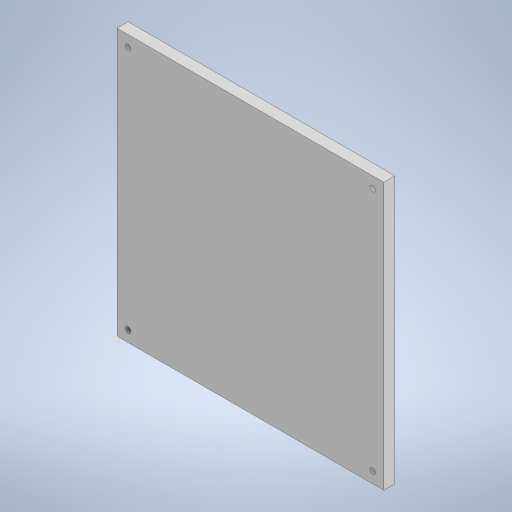
# Autodesk Inventor part: 3d_enclosure_2_19_top_1
Saved by Autodesk Inventor 2024 (Build 280153000, 153)
## iProperties
Created: 2024-02-19
Part Number: 3d_enclosure_2_19_top_1
Material: Generic
Document SubType Name: Modeling
Designer: jtw4137
Density: 1 g/cm^3
Appearance: Default
Author: jtw4137
Autodesk Inventor part; units mm, degrees
ref_plane "YZ Plane" through (0, 0, 0) normal (1, 0, 0) x (0, 1, 0)
ref_plane "XZ Plane" through (0, 0, 0) normal (0, 1, 0) x (-1, 0, 0)
ref_plane "XY Plane" through (0, 0, 0) normal (0, 0, 1) x (1, 0, 0)
sketch "Sketch1" plane through (0, 0, 0) normal (0, 0, 1) x (1, 0, 0)
  line L0 (0, 0) -> (120, 0)
  line L1 (120, 0) -> (120, 120)
  line L2 (120, 120) -> (0, 120)
  line L3 (0, 120) -> (0, 0)
  dimension "d0" = 120
  dimension "d1" = 120
  dimension "d2" = 120
  constraints: 8 end point, 2 perpendicular, 1 horizontal
  measures "d0" distance of L0.start L0.end
  measures "d1" distance of L0.end L1.end
  measures "d2" distance of L1.end L2.end
extrude "Extrusion1" add sketch "Sketch1" along normal blind 5
sketch "Sketch3" plane through (0, 0, 5) normal (0, 0, 1) x (1, 0, 0)
  line L0 (120, 120) -> (0, 120) projected
  line L1 (0, 120) -> (5, 120)
  line L2 (5, 120) -> (5, 115)
  point P0 (0, 0)
  dimension "d7" = 5
  dimension "d8" = 5
  constraints: 4 end point, 1 perpendicular, 1 point on line
  measures "d7" distance of L0.end L1.end
  measures "d8" distance of L1.end L2.end
hole "Hole1" at (5, 115, 5) direction (0, 0, -1) diameter 2.5 depth 38.1 tip angle 118
sketch "Sketch4" plane through (0, 0, 5) normal (0, 0, 1) x (1, 0, 0)
  line L0 (0, 120) -> (0, 0) projected
  line L1 (0, 0) -> (5, 0)
  line L2 (0, 0) -> (120, 0) projected
  line L3 (5, 0) -> (0, 0)
  line L4 (0, 0) -> (0, 5)
  line L5 (0, 5) -> (5, 5)
  dimension "d16" = 5
  dimension "d17" = 5
  dimension "d18" = 5
  dimension "d19" = 5
  constraints: 8 end point, 2 perpendicular, 1 collinear, 1 point on line
  measures "d16" distance of L0.end L1.end
  measures "d17" distance of L1.end L0.end
  measures "d18" distance of L0.end L4.end
  measures "d19" distance of L4.end L5.end
hole "Hole2" at (5, 5, 5) direction (0, 0, -1) diameter 2.5 depth 38.1 tip angle 118
sketch "Sketch8" plane through (0, 0, 5) normal (0, 0, 1) x (1, 0, 0)
  point P0 (0, 0)
sketch "Sketch9" plane through (0, 0, 5) normal (0, 0, 1) x (1, 0, 0)
  line L0 (0, 0) -> (120, 0) projected
  line L1 (120, 0) -> (120, 5)
  line L2 (120, 0) -> (120, 120) projected
  line L3 (120, 5) -> (115, 5)
  dimension "d33" = 5
  dimension "d34" = 5
  constraints: 4 end point, 1 perpendicular, 1 point on line
  measures "d33" distance of L0.end L1.end
  measures "d34" distance of L1.end L3.end
hole "Hole3" at (115, 5, 5) direction (0, 0, -1) diameter 2.5 depth 38.1 tip angle 118
sketch "Sketch10" plane through (0, 0, 5) normal (0, 0, 1) x (1, 0, 0)
  line L0 (120, 120) -> (0, 120) projected
  line L1 (120, 120) -> (120, 115)
  line L2 (120, 0) -> (120, 120) projected
  line L3 (120, 115) -> (115, 115)
  point P0 (0, 0)
  dimension "d42" = 5
  dimension "d43" = 5
  constraints: 4 end point, 1 perpendicular, 1 point on line
  measures "d42" distance of L0.start L1.end
  measures "d43" distance of L1.end L3.end
hole "Hole4" at (115, 115, 5) direction (0, 0, -1) diameter 2.5 depth 38.1 tip angle 118
body "Solid1"
